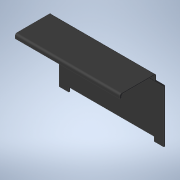
# Autodesk Inventor part: controlbox_cover
Saved by Autodesk Inventor 2020 (Build 240168000, 168)
## iProperties
Created: 2020-06-02
Part Number: controlbox_cover
Material: Generic
Document SubType Name: Modeling
Designer: Gebruiker
Density: 1 g/cm^3
Appearance: Default
Author: Gebruiker
Autodesk Inventor part; units mm, degrees
ref_plane "YZ Plane" through (0, 0, 0) normal (1, 0, 0) x (0, 1, 0)
ref_plane "XZ Plane" through (0, 0, 0) normal (0, 1, 0) x (-1, 0, 0)
ref_plane "XY Plane" through (0, 0, 0) normal (0, 0, 1) x (1, 0, 0)
sketch "Sketch1" plane through (0, 0, 0) normal (1, 0, 0) x (0, 1, 0)
  line L0 (60.5, 1.15) -> (-60.5, 1.15)
  line L1 (-60.5, 1.15) -> (-60.5, -1.15)
  line L2 (-60.5, -1.15) -> (60.5, -1.15)
  line L3 (60.5, -1.15) -> (60.5, 1.15)
  line L4 (60.5, 1.15) -> (-60.5, -1.15) construction
  line L5 (-60.5, 1.15) -> (60.5, -1.15) construction
  line L6 (60.5, -1.15) -> (81.7132, 20.0632)
  line L7 (60.5, -1.15) -> (90.5, -1.15) construction
  line L8 (81.7132, 20.0632) -> (80.0869, 21.6895)
  line L9 (80.0869, 21.6895) -> (59.5288, 1.1315)
  line L10 (80.0869, 21.6895) -> (92.0869, 21.6895)
  line L11 (92.0869, 21.6895) -> (92.0869, 19.3895)
  line L12 (92.0869, 19.3895) -> (81.0395, 19.3895)
  line L13 (92.0869, 19.3895) -> (94.3869, 19.3895)
  line L14 (94.3869, 19.3895) -> (94.3869, 101.3895)
  line L15 (94.3869, 101.3895) -> (92.0869, 101.3895)
  line L16 (92.0869, 101.3895) -> (92.0869, 19.3895)
  line L17 (94.3869, 101.3895) -> (84.3869, 101.3895)
  line L18 (84.3869, 101.3895) -> (84.3869, 97.3895)
  line L19 (84.3869, 97.3895) -> (94.3869, 97.3895)
  line L20 (94.3869, 97.3895) -> (94.3869, 101.3895)
  point P0 (0, 0)
  point P1 (59.5473, 1.15)
  point P2 (92.0869, 97.3895)
  dimension "d0" = 121
  dimension "d1" = 2.3
  dimension "d2" = 30
  dimension "d3" = 45
  dimension "d4" = 2.3
  dimension "d5" = 12
  dimension "d6" = 2.3
  dimension "d7" = 2.3
  dimension "d8" = 82
  dimension "d9" = 10
  dimension "d10" = 4
  constraints: 42 end point, 7 perpendicular, 6 parallel, 5 horizontal, 2 midpoint, 2 point on line, 1 equal length
  measures "d0" distance of L2.end L1.end
  measures "d1" distance of L1.end L0.end
  measures "d2" distance of L2.end L6.end
  measures "d3" angle of L7 L6
  measures "d4" distance of L6.end L8.end
  measures "d5" distance of L8.end L10.end
  measures "d6" distance of L10.end L11.end
  measures "d7" distance of L15.end L14.end
  measures "d8" distance of L14.end L13.end
  measures "d9" distance of L19.end L18.end
  measures "d10" distance of L18.end L17.end
extrude "Extrusion1" add sketch "Sketch1" against normal blind 239
fillet "Fillet1" radius 4 1 edges at (-119.5, 60.5, -1.15)
fillet "Fillet2" radius 4 6 edges at (-119.5, 59.5473, 1.15) (-119.5, 81.0395, 19.3895) (-119.5, 80.0869, 21.6895) (-119.5, 94.3869, 19.3895) (-119.5, 94.3869, 101.3895) (-119.5, 92.0869, 97.3895)
sketch "Sketch2" plane through (0, -60.5, -1.15) normal (0, 0, -1) x (-1, 0, 0)
  line L0 (22, -10) -> (217, -10)
  line L1 (217, -10) -> (217, 10)
  line L2 (217, 10) -> (22, 10)
  line L3 (22, 10) -> (22, -10)
  line L4 (0, 0) -> (239, 0) projected
  line L5 (22, -10) -> (217, 10) construction
  line L6 (217, -10) -> (22, 10) construction
  line L7 (239, 119.3431) -> (239, 0) projected
  line L8 (0, 0) -> (0, 119.3431) projected
  point P0 (0, 60.5)
  point P1 (119.5, 0)
  point P2 (22, 0)
  point P3 (217, 0)
  dimension "d15" = 195
  dimension "d16" = 20
  dimension "d19" = 22
  dimension "d20" = 22
  constraints: 12 end point, 3 midpoint, 2 parallel, 1 horizontal, 1 perpendicular
  measures "d15" distance of L2.end L1.end
  measures "d16" distance of L1.end L0.end
  measures "d19" distance from line of L7 L1.end
  measures "d20" distance from line of L8 L2.end
extrude "Extrusion2" cut sketch "Sketch2" against normal blind 10 contours L3 L2 L1 L4
body "Solid1"
